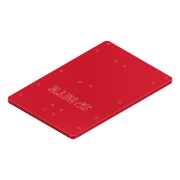
# Autodesk Inventor part: top plate
Saved by Autodesk Inventor 2022 (Build 260153000, 153)
## iProperties
Created: 2024-03-20
Part Number: top plate
Material: Generic
Document SubType Name: Modeling
Designer: david
Density: 1 g/cm^3
Appearance: Smooth - Red
Author: david
Autodesk Inventor part; units mm, degrees
ref_plane "YZ Plane" through (0, 0, 0) normal (1, 0, 0) x (0, 1, 0)
ref_plane "XZ Plane" through (0, 0, 0) normal (0, 1, 0) x (-1, 0, 0)
ref_plane "XY Plane" through (0, 0, 0) normal (0, 0, 1) x (1, 0, 0)
sketch "Sketch1" plane through (0, 0, 0) normal (0, 1, 0) x (-1, 0, 0)
  line L0 (57.5, -173) -> (57.5, -173) construction
  line L1 (-57.5, -173) -> (-57.5, 0) construction
  line L2 (-57.5, 0) -> (57.5, 0)
  line L3 (57.5, 0) -> (57.5, -173) construction
  line L4 (80.5, 0) -> (-80.5, 0) construction
  line L5 (0, -207.6) -> (0, 34.6) construction
  line L6 (57.5, -173) -> (-57.5, -173)
  line L7 (-57.5, -173) -> (-57.5, -173) construction
  line L8 (57.5, 0) -> (-55.1767, 0)
  line L9 (57.5, -40) -> (-57.5, -40) construction
  line L10 (-57.5, -40) -> (-57.5, 0)
  line L11 (-57.5, 0) -> (57.5, 0)
  line L12 (57.5, 0) -> (57.5, -40)
  line L13 (-57.5, -173) -> (-57.5, -40)
  line L14 (57.5, -173) -> (57.5, -40)
  point P0 (0, 0)
  dimension "width" = 115
  dimension "Length" = 173
  dimension "d2" = 115
  dimension "d112" = 40
  constraints: 26 end point, 6 parallel, 5 horizontal, 4 perpendicular, 1 collinear, 1 point on line, 1 symmetric about line, 1 vertical alignment, 1 other
  measures "width" distance of L1.end L2.end
  measures "Length" distance of L1.start L1.end
  measures "d2" distance of L6.end L0.end
  measures "d112" distance between parallel lines of L2 L9
extrude "Base" add sketch "Sketch1" against normal blind 5
sketch "Sketch11" plane through (0, 0, 0) normal (0, 1, 0) x (1, 0, 0)
  line L0 (0, 207.6) -> (0, -34.6) construction
  line L1 (-57.5, 0) -> (57.5, 0) construction
  line L2 (57.5, 173) -> (-57.5, 173) projected
  line L3 (-50, 18) -> (50, 18) construction
  line L4 (50, 18) -> (50, 48) construction
  line L5 (50, 48) -> (-50, 48) construction
  line L6 (-50, 48) -> (-50, 18) construction
  point P0 (0, 0)
  point P1 (50, 168)
  point P2 (-50, 168)
  dimension "d91" = 18
  dimension "d92" = 50
  dimension "d93" = 5
  dimension "d94" = 50
  dimension "d113" = 30
  constraints: 8 end point, 2 coincident, 2 parallel, 2 symmetric about line, 1 horizontal, 1 perpendicular, 1 vertical alignment
  measures "d91" distance from line of L1 point (50, 18)
  measures "d92" distance from line of point (50, 18) L0
  measures "d93" distance from line of L2 point (50, 168)
  measures "d94" distance from line of L0 point (50, 168)
  measures "d113" distance of L3.end L4.end
hole "Mounting Holes" at (50, 0, -18) at (-50, 0, -18) at (50, 0, -168) at (-50, 0, -168) at (-50, 0, -48) at (50, 0, -48) direction (0, -1, 0) diameter 3.4 depth 6
fillet "Fillet1" radius 5 4 edges at (-57.5, -2.5, 0) (57.5, -2.5, -173) (-57.5, -2.5, -173) (57.5, -2.5, 0)
sketch "Sketch12" plane through (0, 0, 0) normal (0, 1, 0) x (1, 0, 0)
  line L0 (-6, 149) -> (43, 149) construction
  line L1 (43, 149) -> (43, 91) construction
  line L2 (43, 91) -> (-6, 91) construction
  line L3 (-6, 91) -> (-6, 149) construction
  line L4 (-57.5, 168) -> (-57.5, 5) projected
  line L5 (0, 207.6) -> (0, -34.6) projected
  line L6 (-52.5, 0) -> (52.5, 0) projected
  circle A0 centre (-50, 48) radius 1.7 projected
  line L7 (52.5, 173) -> (-52.5, 173) projected
  circle A1 centre (50, 48) radius 1.7 projected
  circle A2 centre (50, 168) radius 1.7 projected
  point P0 (0, 0)
  point P1 (0, 0)
  point P2 (52.2987, 0)
  point P3 (-57.5, 40)
  point P4 (0, 0)
  dimension "d104" = 58
  dimension "d263" = 24
  dimension "d266" = 49
  dimension "d267" = 7
  constraints: 8 end point, 1 horizontal, 1 midpoint, 1 parallel, 1 perpendicular, 1 vertical
  measures "d104" distance of L0.end L1.end
  measures "d263" distance between parallel lines of L7 L0
  measures "d266" distance of L1.end L2.end
  measures "d267" distance from line of L1 A2.centre
hole "RasPi Mounting Holes" at (-6, 0, -149) at (43, 0, -149) at (43, 0, -91) at (-6, 0, -91) direction (0, -1, 0) diameter 3.4 depth 6
sketch "Sketch15" plane through (0, 0, 0) normal (0, 1, 0) x (1, 0, 0)
  line L0 (-18, 149) -> (-18, 87.5) construction
  line L1 (-18, 87.5) -> (-50, 87.5) construction
  line L2 (-50, 87.5) -> (-50, 149) construction
  line L3 (-50, 149) -> (-18, 149) construction
  line L4 (-52.5, 0) -> (52.5, 0) projected
  circle A0 centre (43, 149) radius 1.7 projected
  circle A1 centre (50, 48) radius 1.7 projected
  circle A2 centre (-50, 48) radius 1.7 projected
  point P0 (0, 0)
  point P1 (0, 0)
  dimension "d122" = 32
  dimension "d123" = 61.5
  constraints: 8 end point, 4 coincident, 2 parallel, 1 horizontal alignment, 1 midpoint, 1 perpendicular, 1 vertical, 1 vertical alignment
  measures "d122" distance of L2.end L0.start
  measures "d123" distance of L1.end L2.end
hole "LM2596 Mounting Holes" at (-18, 0, -149) at (-18, 0, -87.5) at (-50, 0, -87.5) at (-50, 0, -149) direction (0, -1, 0) diameter 3.4 depth 6
sketch "Sketch16" plane through (0, 0, 0) normal (0, 1, 0) x (1, 0, 0)
  line L0 (-7.5, 16.5) -> (7.5, 16.5) construction
  line L1 (7.5, 16.5) -> (7.5, 30) construction
  line L2 (7.5, 30) -> (-7.5, 30) construction
  line L3 (-7.5, 30) -> (-7.5, 16.5) construction
  line L4 (52.5, 173) -> (-52.5, 173) projected
  line L5 (-52.5, 0) -> (52.5, 0) projected
  point P0 (0, 0)
  point P1 (0, 30)
  point P2 (0, 173)
  dimension "d132" = 15
  dimension "d133" = 13.5
  dimension "d264" = 16.5
  constraints: 8 end point, 4 coincident, 2 midpoint, 2 parallel, 1 horizontal, 1 perpendicular, 1 vertical alignment
  measures "d132" distance of L1.end L2.end
  measures "d133" distance of L2.end L0.start
  measures "d264" distance from line of L5 point (7.5, 16.5)
hole "Camera Mount Mounting Holes" at (-7.5, 0, -30) at (-7.5, 0, -16.5) at (7.5, 0, -16.5) at (7.5, 0, -30) direction (0, -1, 0) diameter 3.4 depth 6
sketch "Sketch17" plane through (0, 0, 0) normal (0, 1, 0) x (1, 0, 0)
  spline S0 degree 4 poles (20.2958, 49.4851) (20.6789, 48.9084) (23.4396, 47.5095) (25.9197, 47.6138) (27.8901, 48.6422) (29.1867, 50.3145) (29.4114, 52.1793) (28.5047, 55.2295) (25.5201, 55.758) (20.7186, 56.8474) (23.8724, 60.2591) (26.3838, 58.5227) (28.1257, 57.2645) knots 0 0 0 0 0 0.20272 0.281354 0.355201 0.433006 0.519581 0.610324 0.697239 0.780233 1 1 1 1 1
  line L0 (28.1257, 57.2645) -> (29.7111, 59.2874)
  line L1 (20.2958, 49.4851) -> (21.6797, 51.6642)
  spline S1 degree 4 poles (21.6797, 51.6642) (22.294, 51.399) (22.8002, 50.5746) (25.5673, 49.8354) (26.8617, 51.423) (26.2496, 52.8197) (24.0458, 53.1534) (23.329, 53.4897) (21.3928, 54.1292) (20.3004, 55.4262) (19.7305, 56.5103) (20.0555, 59.7919) (23.1279, 61.9518) (27.765, 61.4454) (29.2944, 59.5103) (29.7111, 59.2874) knots 0 0 0 0 0 0.144957 0.205265 0.266901 0.324627 0.385746 0.449033 0.50901 0.575778 0.647334 0.728378 0.816759 1 1 1 1 1
  line L2 (19.0392, 48.0812) -> (19.0392, 61.1238)
  line L3 (19.0392, 61.1238) -> (16.3103, 61.1165)
  line L4 (16.3103, 61.1165) -> (16.3103, 57.2645)
  line L5 (16.3005, 50.6209) -> (16.3005, 54.6823)
  line L6 (16.3005, 54.6823) -> (13.9834, 54.6823)
  line L7 (16.3005, 50.6209) -> (13.9834, 50.6209)
  line L8 (19.0392, 48.0812) -> (13.9055, 48.0812)
  line L9 (16.3103, 57.2645) -> (13.9055, 57.2645)
  spline S2 degree 4 poles (13.9055, 48.0812) (12.4379, 47.8667) (9.7187, 48.6838) (8.9871, 53.4702) (10.0145, 55.7471) (11.812, 57.3277) (13.9055, 57.2645) knots 0 0 0 0 0 0.42418 0.584268 1 1 1 1 1
  spline S3 degree 4 poles (13.9834, 50.6209) (12.498, 50.3895) (10.979, 52.4191) (12.1531, 54.6206) (13.9834, 54.6823) knots 0 0 0 0 0 1 1 1 1 1
  line L10 (5.611, 51.8606) -> (5.611, 61.1378)
  line L11 (5.611, 61.1378) -> (2.2951, 61.1378)
  line L12 (2.2951, 61.1378) -> (2.2951, 60.9623)
  line L13 (2.2951, 60.9623) -> (2.2951, 57.2161)
  line L14 (2.2951, 57.2161) -> (0.5839, 57.2161)
  line L15 (0.5839, 57.2161) -> (-1.936, 61.1378)
  line L16 (-1.936, 61.1378) -> (-5.9376, 61.1378)
  line L17 (-5.9376, 61.1378) -> (-3.4177, 57.2161)
  line L18 (5.611, 51.8606) -> (2.2951, 51.8606)
  line L19 (2.2951, 51.8606) -> (2.2951, 53.8306)
  line L20 (2.2951, 53.8306) -> (-1.6405, 53.8306)
  line L21 (-1.6405, 53.8306) -> (-1.6405, 51.2415)
  line L22 (-1.6405, 51.2415) -> (5.611, 51.2415)
  line L23 (5.611, 51.2415) -> (5.611, 47.9336)
  line L24 (5.611, 47.9336) -> (-3.7057, 47.9336)
  line L25 (-5.0121, 49.3829) -> (-5.0121, 55.5531)
  arc A0 (-3.4177, 57.2161) -> (-5.0121, 55.5531) centre (-3.281, 55.4892) ccw
  arc A1 (-5.0121, 49.3829) -> (-3.7057, 47.9336) centre (-2.6718, 50.1788) ccw
  line L26 (-6.9039, 47.9336) -> (-10.2687, 47.9336)
  line L27 (-10.2687, 47.9336) -> (-10.2687, 61.1378)
  line L28 (-10.2687, 61.1378) -> (-6.9039, 61.1378)
  line L29 (-6.9039, 61.1378) -> (-6.9039, 47.9336)
  line L30 (-11.8026, 47.9336) -> (-11.8026, 51.2415)
  line L31 (-11.8026, 51.2415) -> (-15.1713, 51.2415)
  line L32 (-15.1713, 51.2415) -> (-15.1713, 61.1378)
  line L33 (-15.1713, 61.1378) -> (-18.4823, 61.1378)
  line L34 (-18.4823, 61.1378) -> (-18.4823, 47.9336)
  line L35 (-18.4823, 47.9336) -> (-11.8026, 47.9336)
  line L36 (-19.0962, 47.9336) -> (-19.0962, 51.2415)
  line L37 (-19.0962, 51.2415) -> (-21.5406, 51.2415)
  line L38 (-21.5406, 51.2415) -> (-23.787, 47.9336)
  line L39 (-23.787, 47.9336) -> (-19.0962, 47.9336)
  line L40 (-24.4617, 47.9274) -> (-24.4617, 61.1378)
  line L41 (-24.4617, 61.1378) -> (-27.7836, 61.1378)
  line L42 (-27.7836, 61.1378) -> (-27.7836, 47.9274)
  line L43 (-27.7836, 47.9274) -> (-24.4617, 47.9274)
  line L44 (-28.3589, 52.8456) -> (-28.3589, 56.1975)
  line L45 (-28.3589, 56.1975) -> (-30.851, 56.1975)
  line L46 (-30.851, 52.8456) -> (-28.3589, 52.8456)
  line L47 (-27.7836, 47.9274) -> (-27.7836, 51.2654)
  line L48 (-27.7836, 51.2654) -> (-32.8922, 51.2654)
  line L49 (-32.8922, 47.9274) -> (-27.7836, 47.9274)
  line L50 (-32.8922, 47.9274) -> (-35.0606, 51.2654)
  line L51 (-35.0606, 51.2654) -> (-32.8922, 51.2654)
  line L52 (-30.851, 52.8456) -> (-33.0635, 52.8734)
  line L53 (-33.0635, 52.8734) -> (-30.851, 56.1975)
  line L54 (-27.7836, 57.7985) -> (-35.0607, 57.7985)
  line L55 (-35.0607, 57.7985) -> (-32.8922, 61.1378)
  line L56 (-32.8922, 61.1378) -> (-27.7836, 61.1378)
  point P0 (21.8312, 48.4826)
  point P1 (24.6762, 47.7793)
  point P2 (27.8239, 48.7935)
  point P3 (29.2122, 52.0376)
  point P4 (25.048, 55.8974)
  point P5 (22.697, 57.0989)
  point P6 (22.9251, 58.2765)
  point P7 (24.696, 58.9116)
  point P8 (28.2025, 54.5741)
  point P9 (28.8947, 50.19)
  point P10 (26.5311, 48.0478)
  point P11 (22.4682, 51.1588)
  point P12 (23.9337, 50.486)
  point P13 (25.8462, 50.5785)
  point P14 (26.5371, 51.481)
  point P15 (26.0534, 52.5205)
  point P16 (24.2764, 53.1685)
  point P17 (23.1794, 53.5189)
  point P18 (21.5574, 54.2619)
  point P19 (20.447, 55.336)
  point P20 (19.9671, 56.4765)
  point P21 (20.2871, 59.0572)
  point P22 (22.4689, 61.0346)
  point P23 (26.4542, 61.1331)
  point P24 (29.0183, 59.8364)
  point P25 (11.4211, 48.5559)
  point P26 (9.78, 50.5097)
  point P27 (9.4515, 53.0365)
  point P28 (9.8728, 54.8339)
  point P29 (11.0323, 56.3265)
  point P30 (12.7057, 51.0411)
  point P31 (12.0375, 52.3737)
  point P32 (12.4422, 53.8787)
  point P33 (-27.7836, 51.2654)
  point P34 (-3.281, 55.4892)
  constraints: 114 end point, 8 point on line, 4 point on circle, 2 centre point, 41 other
extrude "SP RITE Logo" cut sketch "Sketch17" against normal blind 2 contours L1 S1 L0 S0 | L8 S2 L9 L4 L3 L2 | L7 S3 L6 L5 | L18 L19 L20 L21 L22 L23 L24 A1 L25 A0 L17 L16 L15 L14 L13 L12 L11 L10 | L26 L27 L28 L29 | L35 L34 L33 L32 L31 L30 | L39 L38 L37 L36 | L43 L42 L41 L40 | L49 L50 L51 L48 L42 | L42 L54 L55 L56 | L46 L52 L53 L45 L44
equation "\"d2\" = width"
equation "\"d94\" = d92"
equation "\"d95\" = HoleDia"
equation "\"d105\" = HoleDia"
equation "\"d125\" = HoleDia"
equation "\"d135\" = HoleDia"
equation "\"HoleDia\" = 3.4"
body "Solid1"
